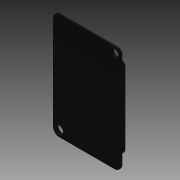
# Autodesk Inventor part: IO-Shield-Sideplate01
Saved by Autodesk Inventor 2013 (Build 170138000, 138)
## iProperties
Created: 2015-02-10
Part Number: IO-Shield-Sideplate01
Material: Generic
Document SubType Name: Modeling
Designer: spichelh
Density: 1 g/cm^3
Author: spichelh
Autodesk Inventor part; units mm, degrees
ref_plane "YZ Plane" through (0, 0, 0) normal (1, 0, 0) x (0, 1, 0)
ref_plane "XZ Plane" through (0, 0, 0) normal (0, 1, 0) x (-1, 0, 0)
ref_plane "XY Plane" through (0, 0, 0) normal (0, 0, 1) x (1, 0, 0)
sketch "Sketch1" plane through (0, 0, 0) normal (0, 0, 1) x (1, 0, 0)
  line L0 (-19.166, -19.1131) -> (-37.166, -19.1131)
  line L1 (-39.166, -17.1131) -> (-39.166, 5.3869)
  line L2 (-37.166, 7.3869) -> (-19.166, 7.3869)
  line L3 (-17.166, 5.3869) -> (-17.166, -17.1131)
  arc A0 (-37.166, 7.3869) -> (-39.166, 5.3869) centre (-37.166, 5.3869) ccw
  arc A1 (-17.166, 5.3869) -> (-19.166, 7.3869) centre (-19.166, 5.3869) ccw
  arc A2 (-19.166, -19.1131) -> (-17.166, -17.1131) centre (-19.166, -17.1131) ccw
  arc A3 (-39.166, -17.1131) -> (-37.166, -19.1131) centre (-37.166, -17.1131) ccw
  point P0 (0, 0)
  dimension "d0" = 2
  dimension "d1" = 22
  dimension "d2" = 26.5
  constraints: 8 end point, 8 point on circle, 8 tangent, 4 centre point, 3 equal radius, 2 parallel, 1 horizontal, 1 perpendicular
  measures "d0" radius of A0
  measures "d1" distance between parallel lines of L1 L3
  measures "d2" distance between parallel lines of L2 L0
extrude "Extrusion1" add sketch "Sketch1" along normal blind 1
sketch "Sketch2" plane through (0, 0, 1) normal (0, 0, 1) x (1, 0, 0)
  line L0 (-39.166, 5.3869) -> (-39.166, -17.1131) projected
  arc A0 (-39.166, -17.1131) -> (-37.166, -19.1131) centre (-37.166, -17.1131) ccw projected
  line L1 (-37.166, -19.1131) -> (-19.166, -19.1131) projected
  arc A1 (-19.166, -19.1131) -> (-17.166, -17.1131) centre (-19.166, -17.1131) ccw projected
  line L2 (-17.166, -17.1131) -> (-17.166, 5.3869) projected
  arc A2 (-17.166, 5.3869) -> (-19.166, 7.3869) centre (-19.166, 5.3869) ccw projected
  line L3 (-19.166, 7.3869) -> (-37.166, 7.3869) projected
  arc A3 (-37.166, 7.3869) -> (-39.166, 5.3869) centre (-37.166, 5.3869) ccw projected
  line L4 (-37.166, 11.3869) -> (-19.166, 11.3869)
  line L5 (-17.166, 9.3869) -> (-17.166, -21.1131)
  line L6 (-19.166, -23.1131) -> (-37.166, -23.1131)
  line L7 (-39.166, -21.1131) -> (-39.166, 9.3869)
  arc A4 (-19.166, -23.1131) -> (-17.166, -21.1131) centre (-19.166, -21.1131) ccw
  arc A5 (-39.166, -21.1131) -> (-37.166, -23.1131) centre (-37.166, -21.1131) ccw
  arc A6 (-37.166, 11.3869) -> (-39.166, 9.3869) centre (-37.166, 9.3869) ccw
  arc A7 (-17.166, 9.3869) -> (-19.166, 11.3869) centre (-19.166, 9.3869) ccw
  circle A8 centre (-37.166, -21.1131) radius 1.25
  circle A9 centre (-19.166, 9.3869) radius 1.25
  point P0 (0, 0)
  dimension "d5" = 2
  dimension "d6" = 4
  dimension "d7" = 4
  dimension "d8" = 2.5
  dimension "d9" = 2.5
  constraints: 8 end point, 8 point on circle, 8 tangent, 6 centre point, 3 equal radius, 2 coincident, 2 collinear, 2 parallel, 1 horizontal, 1 perpendicular
  measures "d5" radius of A4
  measures "d6" distance between parallel lines of L4 L3
  measures "d7" distance between parallel lines of L6 L1
  measures "d8" diameter of A8
  measures "d9" diameter of A9
extrude "Extrusion2" add sketch "Sketch2" along normal blind 1
chamfer "Chamfer1" distance 0.5 angle 45 8 edges at (-38.5802, 6.8011, 0) (-39.166, -5.8631, 0) (-38.5802, -18.5273, 0) (-28.166, -19.1131, 0) (-17.7518, -18.5273, 0) (-17.166, -5.8631, 0) (-17.7518, 6.8011, 0) (-28.166, 7.3869, 0)
chamfer "Chamfer2" distance 0.5 angle 45 10 edges at (-39.166, -19.1131, 1) (-38.5802, -22.5273, 1) (-28.166, -23.1131, 1) (-17.7518, -22.5273, 1) (-17.166, -19.1131, 1) (-39.166, 7.3869, 1) (-38.5802, 10.8011, 1) (-28.166, 11.3869, 1) (-17.7518, 10.8011, 1) (-17.166, 7.3869, 1)
body "Solid1"
